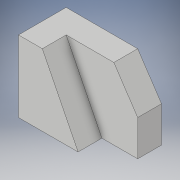
# Autodesk Inventor part: Part9
Saved by Autodesk Inventor 2017 (Build 210142000, 142)
## iProperties
Created: 2016-11-07
Part Number: Part9
Material: Generic
Document SubType Name: Modeling
Designer: s411888
Density: 1 g/cm^3
Appearance: Default
Author: s411888
Autodesk Inventor part; units mm, degrees
ref_plane "YZ Plane" through (0, 0, 0) normal (1, 0, 0) x (0, 1, 0)
ref_plane "XZ Plane" through (0, 0, 0) normal (0, 1, 0) x (-1, 0, 0)
ref_plane "XY Plane" through (0, 0, 0) normal (0, 0, 1) x (1, 0, 0)
sketch "Sketch1" plane through (0, 0, 0) normal (0, 0, 1) x (1, 0, 0)
  line L0 (-25.6265, 18.4793) -> (25.1735, 18.4793)
  line L1 (25.1735, 18.4793) -> (25.1735, -19.6207)
  line L2 (25.1735, -19.6207) -> (-25.6265, -19.6207)
  line L3 (-25.6265, -19.6207) -> (-25.6265, 18.4793)
  point P0 (0, 0)
  dimension "d0" = 50.8
  dimension "d1" = 38.1
  constraints: 8 end point, 2 parallel, 1 horizontal, 1 perpendicular
  measures "d0" distance of L1.end L2.end
  measures "d1" distance of L0.end L1.end
extrude "Extrusion1" add sketch "Sketch1" along normal blind 25.4
sketch "Sketch2" plane through (0, 0, 25.4) normal (0, 0, 1) x (1, 0, 0)
  line L0 (25.1735, 18.4793) -> (-25.6265, 18.4793) projected
  line L1 (25.1735, 18.4793) -> (25.1735, -0.5707)
  line L2 (25.1735, -19.6207) -> (25.1735, 18.4793) projected
  line L3 (25.1735, 18.4793) -> (12.4735, 18.4793)
  line L4 (12.4735, 18.4793) -> (25.1735, -0.5707)
  line L5 (-25.6265, 18.4793) -> (-12.9265, 18.4793)
  line L6 (25.1735, -19.6207) -> (6.1235, -19.6207)
  line L7 (-25.6265, -19.6207) -> (25.1735, -19.6207) projected
  line L8 (6.1235, -19.6207) -> (-12.9265, 18.4793)
  line L9 (-12.9265, 18.4793) -> (12.4735, 18.4793)
  line L10 (25.1735, -0.5707) -> (25.1735, -19.6207)
  point P0 (0, 0)
  dimension "d4" = 19.05
  dimension "d5" = 12.7
  dimension "d6" = 12.7
  dimension "d7" = 19.05
  constraints: 16 end point, 3 point on line, 1 collinear, 1 midpoint, 1 perpendicular
  measures "d4" distance of L0.start L1.end
  measures "d5" distance of L0.start L3.end
  measures "d6" distance of L0.end L5.end
  measures "d7" distance of L2.start L6.end
extrude "Extrusion2" cut sketch "Sketch2" against normal blind 25.4 contours L1 L4 L0
extrude "Extrusion3" cut sketch "Sketch2" against normal blind 12.7 contours L4 L2 L6 L8 L0
body "Solid1"
